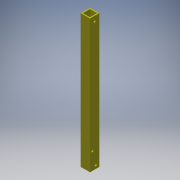
# Autodesk Inventor part: cylinder arm
Saved by Autodesk Inventor 2017 SP1 (Build 210196100, 196)
## iProperties
Created: 2018-01-27
Part Number: cylinder arm
Material: Aluminum 6061
Document SubType Name: Modeling
Designer: Ben
Density: 2.7 g/cm^3
Appearance: Canary
Author: Ben
Autodesk Inventor part; units mm, degrees
ref_plane "YZ Plane" through (0, 0, 0) normal (1, 0, 0) x (0, 1, 0)
ref_plane "XZ Plane" through (0, 0, 0) normal (0, 1, 0) x (-1, 0, 0)
ref_plane "XY Plane" through (0, 0, 0) normal (0, 0, 1) x (1, 0, 0)
sketch "Sketch1" plane through (0, 0, 0) normal (0, 1, 0) x (-1, 0, 0)
  line L0 (-12.7, 12.7) -> (12.7, 12.7)
  line L1 (12.7, 12.7) -> (12.7, -12.7)
  line L2 (12.7, -12.7) -> (-12.7, -12.7)
  line L3 (-12.7, -12.7) -> (-12.7, 12.7)
  line L4 (-12.7, 12.7) -> (12.7, -12.7) construction
  line L5 (12.7, 12.7) -> (-12.7, -12.7) construction
  line L6 (-9.525, 9.525) -> (9.525, 9.525)
  line L7 (9.525, 9.525) -> (9.525, -9.525)
  line L8 (9.525, -9.525) -> (-9.525, -9.525)
  line L9 (-9.525, -9.525) -> (-9.525, 9.525)
  line L10 (-9.525, 9.525) -> (9.525, -9.525) construction
  line L11 (9.525, 9.525) -> (-9.525, -9.525) construction
  point P0 (0, 0)
  dimension "d0" = 25.4
  dimension "d1" = 3.175
  constraints: 24 end point, 4 midpoint, 4 parallel, 3 perpendicular, 2 horizontal, 1 point on line
  measures "d0" distance of L1.end L2.end
  measures "d1" distance between parallel lines of L2 L8
extrude "Extrusion1" add sketch "Sketch1" along normal mid plane 361.95
sketch "Sketch2" plane through (12.7, -180.975, -12.7) normal (1, 0, 0) x (0, 0, -1)
  line L0 (0, 0) -> (-25.4, 0) construction
  line L1 (-25.4, 361.95) -> (0, 361.95) construction
  circle A0 centre (-15.875, -13.0676) radius 3.302 construction
  circle A1 centre (-19.05, 47.1738) radius 3.302
  circle A2 centre (-9.486, 9.525) radius 3.302
  circle A3 centre (-12.7, 349.1893) radius 3.302
  line L2 (-15.875, -13.0676) -> (-19.05, 47.1738) construction
  line L3 (-25.4, 0) -> (-25.4, 361.95) construction
  line L4 (-3.175, 361.95) -> (-3.175, 0) construction
  line L5 (-9.486, 15.9408) -> (-3.9298, 12.7329)
  line L6 (-3.9298, 12.7329) -> (-3.9298, 6.3171)
  line L7 (-3.9298, 6.3171) -> (-9.486, 3.1092)
  line L8 (-9.486, 3.1092) -> (-15.0423, 6.3171)
  line L9 (-15.0423, 6.3171) -> (-15.0423, 12.7329)
  line L10 (-15.0423, 12.7329) -> (-9.486, 15.9408)
  line L11 (-9.486, 9.525) -> (-11.4913, 47.5722) construction
  line L12 (-11.4913, 47.5722) -> (-19.05, 47.1738) construction
  point P0 (-12.7, 180.975)
  dimension "d5" = 6.604
  dimension "d6" = 60.325
  dimension "d9" = 6.604
  dimension "d10" = 302.0822
  dimension "d14" = 6.35
  dimension "d15" = 7.5692
  dimension "d16" = 12.7
  dimension "d17" = 6.604
  dimension "d18" = 11.1125
  dimension "d19" = 3.017
  dimension "d20" = 9.525
  dimension "d22" = 38.1
  constraints: 18 end point, 4 centre point, 2 parallel, 1 coincident, 1 equal radius, 1 perpendicular, 13 other
  measures "d5" diameter of A0
  measures "d6" distance of L2.start L2.end
  measures "d9" diameter of A3
  measures "d10" distance of L2.end A3.centre
  measures "d14" distance from line of L3 L2.end
  measures "d15" distance from line of L2 A2.centre
  measures "d16" distance from line of L3 A3.centre
  measures "d17" diameter of A2
  measures "d18" distance between parallel lines of L9 L6
  measures "d19" angle of L3 L2
  measures "d20" distance from line of L0 A2.centre
  measures "d22" distance of L11.start L11.end
extrude "Extrusion2" cut sketch "Sketch2" against normal through all contours A1 | A2 | A3
body "Solid1"
